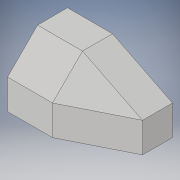
# Autodesk Inventor part: 零件13
Saved by Autodesk Inventor 2019 (Build 230136000, 136)
## iProperties
Created: 2020-09-18
Part Number: 零件13
Material: 一般
Document SubType Name: Modeling
Designer: jay
Density: 1 g/cm^3
Appearance: 預設
Author: jay
Autodesk Inventor part; units mm, degrees
ref_plane "YZ Plane" through (0, 0, 0) normal (1, 0, 0) x (0, 1, 0)
ref_plane "XZ Plane" through (0, 0, 0) normal (0, 1, 0) x (-1, 0, 0)
sketch "草圖5" plane through (0, 0, 0) normal (0, 0, 1) x (1, 0, 0)
  line L0 (0, 0) -> (70, 0)
  line L1 (70, 0) -> (70, 40)
  line L2 (70, 40) -> (0, 40)
  line L3 (0, 40) -> (0, 0)
  dimension "d20" = 70
  dimension "d21" = 40
  constraints: 8 end point, 2 parallel, 1 horizontal, 1 perpendicular
  measures "d20" distance of L1.end L2.end
  measures "d21" distance of L0.end L1.end
extrude "擠出5" add sketch "草圖5" along normal blind 40
chamfer "倒角2" distance 20 distance2 40 1 edges at (70, 40, 20) measured on face at (70, 13.3333, 13.3333)
chamfer "倒角3" distance 20 distance2 20 1 edges at (15, 40, 40) measured on face at (33.3333, 13.3333, 40)
chamfer "倒角4" distance 40 distance2 20 1 edges at (70, 10, 40) measured on face at (23.3333, 13.3333, 40)
ref_plane "工作平面1" through (70, 20, 20) normal (0.3333, 0.6667, 0.6667) x (-0.8944, 0.4472, 0)
sketch "草圖9" plane through (70, 20, 20) normal (0.3333, 0.6667, 0.6667) x (-0.8944, 0.4472, 0)
  point P0 (53.6656, 17.8885)
sketch "草圖10" plane through (70, 20, 20) normal (0.3333, 0.6667, 0.6667) x (-0.8944, 0.4472, 0)
  line L0 (44.7214, -14.9071) -> (44.7214, 0) projected
  line L1 (44.7214, 0) -> (0, 0)
  line L2 (53.6656, 17.8885) -> (-8.9443, -2.9814) projected
  line L3 (0, 0) -> (35.7302, 26.9735)
  line L4 (44.7214, 0) -> (71.5542, 8.9443) projected
  line L5 (35.7302, 26.9735) -> (44.7214, 0)
  constraints: 6 end point, 1 horizontal, 1 perpendicular, 1 point on line
extrude "擠出8" cut sketch "草圖10" along normal through all
